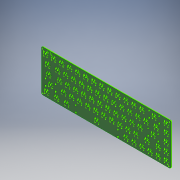
# Autodesk Inventor part: 60pc_pcb.kicad_pcb_Outline
Saved by Autodesk Inventor 2018 (Build 220112000, 112)
## iProperties
Created: 2018-02-01
Part Number: 60pc_pcb.kicad_pcb_Outline
Material: Generic
Document SubType Name: Modeling
Designer: ConnorDevitt
Density: 1 g/cm^3
Appearance: Board Outline
Author: ConnorDevitt
Autodesk Inventor part; units mm, degrees
(part 1 of 2)
ref_plane "YZ Plane" through (0, 0, 0) normal (1, 0, 0) x (0, 1, 0)
ref_plane "XZ Plane" through (0, 0, 0) normal (0, 1, 0) x (-1, 0, 0)
ref_plane "XY Plane" through (0, 0, 0) normal (0, 0, 1) x (1, 0, 0)
sketch "Sketch1" plane through (0, 0, 0) normal (0, 0, 1) x (1, 0, 0)
  arc A0 (77.75, -126.75) -> (81.75, -130.75) centre (81.75, -126.75) ccw
  line L0 (81.75, -130.75) -> (380.25, -130.75)
  arc A1 (380.25, -130.75) -> (384.25, -126.75) centre (380.25, -126.75) ccw
  line L1 (384.25, -126.75) -> (384.25, -35.25)
  arc A2 (384.25, -35.25) -> (381.5, -32.5) centre (381.5, -35.25) ccw
  line L2 (381.5, -32.5) -> (80.5, -32.5)
  arc A3 (80.5, -32.5) -> (77.75, -35.25) centre (80.5, -35.25) ccw
  line L3 (77.75, -35.25) -> (77.75, -126.75)
  line L4 (104.8123, -39.2267) -> (104.0014, -40.6866)
  arc A4 (102.6902, -39.9583) -> (104.0014, -40.6866) centre (103.3458, -40.3225) ccw
  line L5 (102.6902, -39.9583) -> (103.5011, -38.4984)
  arc A5 (104.8123, -39.2267) -> (103.5011, -38.4984) centre (104.1567, -38.8625) ccw
  line L6 (110.4442, -37.8342) -> (110.4048, -38.4128)
  arc A6 (108.9083, -38.3108) -> (110.4048, -38.4128) centre (109.6565, -38.3618) ccw
  line L7 (108.9083, -38.3108) -> (108.9477, -37.7322)
  arc A7 (110.4442, -37.8342) -> (108.9477, -37.7322) centre (109.696, -37.7832) ccw
  line L8 (94.49, -34.45) -> (94.49, -36.95)
  arc A8 (93.79, -36.95) -> (94.49, -36.95) centre (94.14, -36.95) ccw
  line L9 (93.79, -36.95) -> (93.79, -34.45)
  arc A9 (94.49, -34.45) -> (93.79, -34.45) centre (94.14, -34.45) ccw
  line L10 (101.79, -34.45) -> (101.79, -36.95)
  arc A10 (101.09, -36.95) -> (101.79, -36.95) centre (101.44, -36.95) ccw
  line L11 (101.09, -36.95) -> (101.09, -34.45)
  arc A11 (101.79, -34.45) -> (101.09, -34.45) centre (101.44, -34.45) ccw
  line L12 (85.7623, -39.2267) -> (84.9514, -40.6866)
  arc A12 (83.6402, -39.9583) -> (84.9514, -40.6866) centre (84.2958, -40.3225) ccw
  line L13 (83.6402, -39.9583) -> (84.4511, -38.4984)
  arc A13 (85.7623, -39.2267) -> (84.4511, -38.4984) centre (85.1067, -38.8625) ccw
  line L14 (91.3942, -37.8342) -> (91.3548, -38.4128)
  arc A14 (89.8583, -38.3108) -> (91.3548, -38.4128) centre (90.6065, -38.3618) ccw
  line L15 (89.8583, -38.3108) -> (89.8977, -37.7322)
  arc A15 (91.3942, -37.8342) -> (89.8977, -37.7322) centre (90.646, -37.7832) ccw
  line L16 (90.5249, -58.2767) -> (89.7139, -59.7366)
  arc A16 (88.4027, -59.0083) -> (89.7139, -59.7366) centre (89.0583, -59.3725) ccw
  line L17 (88.4027, -59.0083) -> (89.2136, -57.5484)
  arc A17 (90.5249, -58.2767) -> (89.2136, -57.5484) centre (89.8692, -57.9125) ccw
  line L18 (96.1567, -56.8842) -> (96.1173, -57.4628)
  arc A18 (94.6208, -57.3608) -> (96.1173, -57.4628) centre (95.369, -57.4118) ccw
  line L19 (94.6208, -57.3608) -> (94.6602, -56.7822)
  arc A19 (96.1567, -56.8842) -> (94.6602, -56.7822) centre (95.4085, -56.8332) ccw
  line L20 (92.9061, -77.3267) -> (92.0952, -78.7866)
  arc A20 (90.7839, -78.0583) -> (92.0952, -78.7866) centre (91.4395, -78.4225) ccw
  line L21 (90.7839, -78.0583) -> (91.5948, -76.5984)
  arc A21 (92.9061, -77.3267) -> (91.5948, -76.5984) centre (92.2505, -76.9625) ccw
  line L22 (98.538, -75.9342) -> (98.4985, -76.5128)
  arc A22 (97.002, -76.4108) -> (98.4985, -76.5128) centre (97.7503, -76.4618) ccw
  line L23 (97.002, -76.4108) -> (97.0415, -75.8322)
  arc A23 (98.538, -75.9342) -> (97.0415, -75.8322) centre (97.7897, -75.8832) ccw
  line L24 (97.6686, -96.3767) -> (96.8577, -97.8366)
  arc A24 (95.5464, -97.1083) -> (96.8577, -97.8366) centre (96.202, -97.4725) ccw
  line L25 (95.5464, -97.1083) -> (96.3573, -95.6484)
  arc A25 (97.6686, -96.3767) -> (96.3573, -95.6484) centre (97.013, -96.0125) ccw
  line L26 (103.3005, -94.9842) -> (103.261, -95.5628)
  arc A26 (101.7645, -95.4608) -> (103.261, -95.5628) centre (102.5128, -95.5118) ccw
  line L27 (101.7645, -95.4608) -> (101.804, -94.8822)
  arc A27 (103.3005, -94.9842) -> (101.804, -94.8822) centre (102.5522, -94.9332) ccw
  line L28 (88.1436, -115.4267) -> (87.3327, -116.8866)
  arc A28 (86.0214, -116.1583) -> (87.3327, -116.8866) centre (86.677, -116.5225) ccw
  line L29 (86.0214, -116.1583) -> (86.8323, -114.6984)
  arc A29 (88.1436, -115.4267) -> (86.8323, -114.6984) centre (87.488, -115.0625) ccw
  line L30 (93.7755, -114.0342) -> (93.736, -114.6128)
  arc A30 (92.2395, -114.5108) -> (93.736, -114.6128) centre (92.9878, -114.5618) ccw
  line L31 (92.2395, -114.5108) -> (92.279, -113.9322)
  arc A31 (93.7755, -114.0342) -> (92.279, -113.9322) centre (93.0272, -113.9832) ccw
  line L32 (114.3374, -58.2767) -> (113.5264, -59.7366)
  arc A32 (112.2151, -59.0083) -> (113.5264, -59.7366) centre (112.8708, -59.3725) ccw
  line L33 (112.2151, -59.0083) -> (113.0261, -57.5484)
  arc A33 (114.3374, -58.2767) -> (113.0261, -57.5484) centre (113.6817, -57.9125) ccw
  line L34 (119.9692, -56.8842) -> (119.9298, -57.4628)
  arc A34 (118.4333, -57.3608) -> (119.9298, -57.4628) centre (119.1815, -57.4118) ccw
  line L35 (118.4333, -57.3608) -> (118.4727, -56.7822)
  arc A35 (119.9692, -56.8842) -> (118.4727, -56.7822) centre (119.221, -56.8332) ccw
  line L36 (119.0999, -77.3267) -> (118.2889, -78.7866)
  arc A36 (116.9777, -78.0583) -> (118.2889, -78.7866) centre (117.6333, -78.4225) ccw
  line L37 (116.9777, -78.0583) -> (117.7886, -76.5984)
  arc A37 (119.0999, -77.3267) -> (117.7886, -76.5984) centre (118.4442, -76.9625) ccw
  line L38 (124.7317, -75.9342) -> (124.6923, -76.5128)
  arc A38 (123.1958, -76.4108) -> (124.6923, -76.5128) centre (123.944, -76.4618) ccw
  line L39 (123.1958, -76.4108) -> (123.2352, -75.8322)
  arc A39 (124.7317, -75.9342) -> (123.2352, -75.8322) centre (123.9835, -75.8832) ccw
  line L40 (128.6249, -96.3767) -> (127.8139, -97.8366)
  arc A40 (126.5027, -97.1083) -> (127.8139, -97.8366) centre (127.1583, -97.4725) ccw
  line L41 (126.5027, -97.1083) -> (127.3136, -95.6484)
  arc A41 (128.6249, -96.3767) -> (127.3136, -95.6484) centre (127.9692, -96.0125) ccw
  line L42 (134.2567, -94.9842) -> (134.2173, -95.5628)
  arc A42 (132.7208, -95.4608) -> (134.2173, -95.5628) centre (133.469, -95.5118) ccw
  line L43 (132.7208, -95.4608) -> (132.7602, -94.8822)
  arc A43 (134.2567, -94.9842) -> (132.7602, -94.8822) centre (133.5085, -94.9332) ccw
  line L44 (111.9561, -115.4267) -> (111.1452, -116.8866)
  arc A44 (109.8339, -116.1583) -> (111.1452, -116.8866) centre (110.4895, -116.5225) ccw
  line L45 (109.8339, -116.1583) -> (110.6448, -114.6984)
  arc A45 (111.9561, -115.4267) -> (110.6448, -114.6984) centre (111.3005, -115.0625) ccw
  line L46 (117.588, -114.0342) -> (117.5485, -114.6128)
  arc A46 (116.052, -114.5108) -> (117.5485, -114.6128) centre (116.8003, -114.5618) ccw
  line L47 (116.052, -114.5108) -> (116.0915, -113.9322)
  arc A47 (117.588, -114.0342) -> (116.0915, -113.9322) centre (116.8397, -113.9832) ccw
  line L48 (135.7686, -115.4267) -> (134.9577, -116.8866)
  arc A48 (133.6464, -116.1583) -> (134.9577, -116.8866) centre (134.302, -116.5225) ccw
  line L49 (133.6464, -116.1583) -> (134.4573, -114.6984)
  arc A49 (135.7686, -115.4267) -> (134.4573, -114.6984) centre (135.113, -115.0625) ccw
  line L50 (141.4005, -114.0342) -> (141.361, -114.6128)
  arc A50 (139.8645, -114.5108) -> (141.361, -114.6128) centre (140.6128, -114.5618) ccw
  line L51 (139.8645, -114.5108) -> (139.904, -113.9322)
  arc A51 (141.4005, -114.0342) -> (139.904, -113.9322) centre (140.6522, -113.9832) ccw
  line L52 (123.8624, -39.2267) -> (123.0514, -40.6866)
  arc A52 (121.7401, -39.9583) -> (123.0514, -40.6866) centre (122.3958, -40.3225) ccw
  line L53 (121.7401, -39.9583) -> (122.5511, -38.4984)
  arc A53 (123.8624, -39.2267) -> (122.5511, -38.4984) centre (123.2067, -38.8625) ccw
  line L54 (129.4942, -37.8342) -> (129.4548, -38.4128)
  arc A54 (127.9583, -38.3108) -> (129.4548, -38.4128) centre (128.7065, -38.3618) ccw
  line L55 (127.9583, -38.3108) -> (127.9977, -37.7322)
  arc A55 (129.4942, -37.8342) -> (127.9977, -37.7322) centre (128.746, -37.7832) ccw
  line L56 (133.3873, -58.2767) -> (132.5764, -59.7366)
  arc A56 (131.2652, -59.0083) -> (132.5764, -59.7366) centre (131.9208, -59.3725) ccw
  line L57 (131.2652, -59.0083) -> (132.0761, -57.5484)
  arc A57 (133.3873, -58.2767) -> (132.0761, -57.5484) centre (132.7317, -57.9125) ccw
  line L58 (139.0192, -56.8842) -> (138.9798, -57.4628)
  arc A58 (137.4833, -57.3608) -> (138.9798, -57.4628) centre (138.2315, -57.4118) ccw
  line L59 (137.4833, -57.3608) -> (137.5227, -56.7822)
  arc A59 (139.0192, -56.8842) -> (137.5227, -56.7822) centre (138.271, -56.8332) ccw
  line L60 (138.1499, -77.3267) -> (137.3389, -78.7866)
  arc A60 (136.0276, -78.0583) -> (137.3389, -78.7866) centre (136.6833, -78.4225) ccw
  line L61 (136.0276, -78.0583) -> (136.8386, -76.5984)
  arc A61 (138.1499, -77.3267) -> (136.8386, -76.5984) centre (137.4942, -76.9625) ccw
  line L62 (143.7817, -75.9342) -> (143.7423, -76.5128)
  arc A62 (142.2458, -76.4108) -> (143.7423, -76.5128) centre (142.994, -76.4618) ccw
  line L63 (142.2458, -76.4108) -> (142.2852, -75.8322)
  arc A63 (143.7817, -75.9342) -> (142.2852, -75.8322) centre (143.0335, -75.8832) ccw
  line L64 (147.6748, -96.3767) -> (146.8639, -97.8366)
  arc A64 (145.5526, -97.1083) -> (146.8639, -97.8366) centre (146.2083, -97.4725) ccw
  line L65 (145.5526, -97.1083) -> (146.3636, -95.6484)
  arc A65 (147.6748, -96.3767) -> (146.3636, -95.6484) centre (147.0192, -96.0125) ccw
  line L66 (153.3067, -94.9842) -> (153.2673, -95.5628)
  arc A66 (151.7708, -95.4608) -> (153.2673, -95.5628) centre (152.519, -95.5118) ccw
  line L67 (151.7708, -95.4608) -> (151.8102, -94.8822)
  arc A67 (153.3067, -94.9842) -> (151.8102, -94.8822) centre (152.5585, -94.9332) ccw
  line L68 (142.9124, -39.2267) -> (142.1014, -40.6866)
  arc A68 (140.7902, -39.9583) -> (142.1014, -40.6866) centre (141.4458, -40.3225) ccw
  line L69 (140.7902, -39.9583) -> (141.6011, -38.4984)
  arc A69 (142.9124, -39.2267) -> (141.6011, -38.4984) centre (142.2567, -38.8625) ccw
  line L70 (148.5442, -37.8342) -> (148.5048, -38.4128)
  arc A70 (147.0083, -38.3108) -> (148.5048, -38.4128) centre (147.7565, -38.3618) ccw
  line L71 (147.0083, -38.3108) -> (147.0477, -37.7322)
  arc A71 (148.5442, -37.8342) -> (147.0477, -37.7322) centre (147.796, -37.7832) ccw
  line L72 (152.4374, -58.2767) -> (151.6264, -59.7366)
  arc A72 (150.3151, -59.0083) -> (151.6264, -59.7366) centre (150.9708, -59.3725) ccw
  line L73 (150.3151, -59.0083) -> (151.1261, -57.5484)
  arc A73 (152.4374, -58.2767) -> (151.1261, -57.5484) centre (151.7817, -57.9125) ccw
  line L74 (158.0692, -56.8842) -> (158.0298, -57.4628)
  arc A74 (156.5333, -57.3608) -> (158.0298, -57.4628) centre (157.2815, -57.4118) ccw
  line L75 (156.5333, -57.3608) -> (156.5727, -56.7822)
  arc A75 (158.0692, -56.8842) -> (156.5727, -56.7822) centre (157.321, -56.8332) ccw
  line L76 (157.1999, -77.3267) -> (156.3889, -78.7866)
  arc A76 (155.0777, -78.0583) -> (156.3889, -78.7866) centre (155.7333, -78.4225) ccw
  line L77 (155.0777, -78.0583) -> (155.8886, -76.5984)
  arc A77 (157.1999, -77.3267) -> (155.8886, -76.5984) centre (156.5442, -76.9625) ccw
  line L78 (162.8317, -75.9342) -> (162.7923, -76.5128)
  arc A78 (161.2958, -76.4108) -> (162.7923, -76.5128) centre (162.044, -76.4618) ccw
  line L79 (161.2958, -76.4108) -> (161.3352, -75.8322)
  arc A79 (162.8317, -75.9342) -> (161.3352, -75.8322) centre (162.0835, -75.8832) ccw
  line L80 (166.7249, -96.3767) -> (165.9139, -97.8366)
  arc A80 (164.6027, -97.1083) -> (165.9139, -97.8366) centre (165.2583, -97.4725) ccw
  line L81 (164.6027, -97.1083) -> (165.4136, -95.6484)
  arc A81 (166.7249, -96.3767) -> (165.4136, -95.6484) centre (166.0692, -96.0125) ccw
  line L82 (172.3567, -94.9842) -> (172.3173, -95.5628)
  arc A82 (170.8208, -95.4608) -> (172.3173, -95.5628) centre (171.569, -95.5118) ccw
  line L83 (170.8208, -95.4608) -> (170.8602, -94.8822)
  arc A83 (172.3567, -94.9842) -> (170.8602, -94.8822) centre (171.6085, -94.9332) ccw
  line L84 (161.9623, -39.2267) -> (161.1514, -40.6866)
  arc A84 (159.8401, -39.9583) -> (161.1514, -40.6866) centre (160.4958, -40.3225) ccw
  line L85 (159.8401, -39.9583) -> (160.6511, -38.4984)
  arc A85 (161.9623, -39.2267) -> (160.6511, -38.4984) centre (161.3067, -38.8625) ccw
  line L86 (167.5942, -37.8342) -> (167.5548, -38.4128)
  arc A86 (166.0583, -38.3108) -> (167.5548, -38.4128) centre (166.8065, -38.3618) ccw
  line L87 (166.0583, -38.3108) -> (166.0977, -37.7322)
  arc A87 (167.5942, -37.8342) -> (166.0977, -37.7322) centre (166.846, -37.7832) ccw
  line L88 (171.4873, -58.2767) -> (170.6764, -59.7366)
  arc A88 (169.3651, -59.0083) -> (170.6764, -59.7366) centre (170.0208, -59.3725) ccw
  line L89 (169.3651, -59.0083) -> (170.1761, -57.5484)
  arc A89 (171.4873, -58.2767) -> (170.1761, -57.5484) centre (170.8317, -57.9125) ccw
  line L90 (177.1192, -56.8842) -> (177.0798, -57.4628)
  arc A90 (175.5833, -57.3608) -> (177.0798, -57.4628) centre (176.3315, -57.4118) ccw
  line L91 (175.5833, -57.3608) -> (175.6227, -56.7822)
  arc A91 (177.1192, -56.8842) -> (175.6227, -56.7822) centre (176.371, -56.8332) ccw
  line L92 (176.2499, -77.3267) -> (175.4389, -78.7866)
  arc A92 (174.1277, -78.0583) -> (175.4389, -78.7866) centre (174.7833, -78.4225) ccw
  line L93 (174.1277, -78.0583) -> (174.9386, -76.5984)
  arc A93 (176.2499, -77.3267) -> (174.9386, -76.5984) centre (175.5942, -76.9625) ccw
  line L94 (181.8817, -75.9342) -> (181.8423, -76.5128)
  arc A94 (180.3458, -76.4108) -> (181.8423, -76.5128) centre (181.094, -76.4618) ccw
  line L95 (180.3458, -76.4108) -> (180.3852, -75.8322)
  arc A95 (181.8817, -75.9342) -> (180.3852, -75.8322) centre (181.1335, -75.8832) ccw
  line L96 (185.7748, -96.3767) -> (184.9639, -97.8366)
  arc A96 (183.6526, -97.1083) -> (184.9639, -97.8366) centre (184.3083, -97.4725) ccw
  line L97 (183.6526, -97.1083) -> (184.4636, -95.6484)
  arc A97 (185.7748, -96.3767) -> (184.4636, -95.6484) centre (185.1192, -96.0125) ccw
  line L98 (191.4067, -94.9842) -> (191.3673, -95.5628)
  arc A98 (189.8708, -95.4608) -> (191.3673, -95.5628) centre (190.619, -95.5118) ccw
  line L99 (189.8708, -95.4608) -> (189.9102, -94.8822)
  arc A99 (191.4067, -94.9842) -> (189.9102, -94.8822) centre (190.6585, -94.9332) ccw
  line L100 (181.0123, -39.2267) -> (180.2014, -40.6866)
  arc A100 (178.8902, -39.9583) -> (180.2014, -40.6866) centre (179.5458, -40.3225) ccw
  line L101 (178.8902, -39.9583) -> (179.7011, -38.4984)
  arc A101 (181.0123, -39.2267) -> (179.7011, -38.4984) centre (180.3567, -38.8625) ccw
  line L102 (186.6442, -37.8342) -> (186.6048, -38.4128)
  arc A102 (185.1083, -38.3108) -> (186.6048, -38.4128) centre (185.8565, -38.3618) ccw
  line L103 (185.1083, -38.3108) -> (185.1477, -37.7322)
  arc A103 (186.6442, -37.8342) -> (185.1477, -37.7322) centre (185.896, -37.7832) ccw
  line L104 (190.5374, -58.2767) -> (189.7264, -59.7366)
  arc A104 (188.4152, -59.0083) -> (189.7264, -59.7366) centre (189.0708, -59.3725) ccw
  line L105 (188.4152, -59.0083) -> (189.2261, -57.5484)
  arc A105 (190.5374, -58.2767) -> (189.2261, -57.5484) centre (189.8817, -57.9125) ccw
  line L106 (196.1692, -56.8842) -> (196.1298, -57.4628)
  arc A106 (194.6333, -57.3608) -> (196.1298, -57.4628) centre (195.3815, -57.4118) ccw
  line L107 (194.6333, -57.3608) -> (194.6727, -56.7822)
  arc A107 (196.1692, -56.8842) -> (194.6727, -56.7822) centre (195.421, -56.8332) ccw
  line L108 (195.2998, -77.3267) -> (194.4889, -78.7866)
  arc A108 (193.1777, -78.0583) -> (194.4889, -78.7866) centre (193.8333, -78.4225) ccw
  line L109 (193.1777, -78.0583) -> (193.9886, -76.5984)
  arc A109 (195.2998, -77.3267) -> (193.9886, -76.5984) centre (194.6442, -76.9625) ccw
  line L110 (200.9317, -75.9342) -> (200.8923, -76.5128)
  arc A110 (199.3958, -76.4108) -> (200.8923, -76.5128) centre (200.144, -76.4618) ccw
  line L111 (199.3958, -76.4108) -> (199.4352, -75.8322)
  arc A111 (200.9317, -75.9342) -> (199.4352, -75.8322) centre (200.1835, -75.8832) ccw
  line L112 (204.8248, -96.3767) -> (204.0139, -97.8366)
  arc A112 (202.7027, -97.1083) -> (204.0139, -97.8366) centre (203.3583, -97.4725) ccw
  line L113 (202.7027, -97.1083) -> (203.5136, -95.6484)
  arc A113 (204.8248, -96.3767) -> (203.5136, -95.6484) centre (204.1692, -96.0125) ccw
  line L114 (210.4567, -94.9842) -> (210.4173, -95.5628)
  arc A114 (208.9208, -95.4608) -> (210.4173, -95.5628) centre (209.669, -95.5118) ccw
  line L115 (208.9208, -95.4608) -> (208.9602, -94.8822)
  arc A115 (210.4567, -94.9842) -> (208.9602, -94.8822) centre (209.7085, -94.9332) ccw
  line L116 (200.0624, -39.2267) -> (199.2514, -40.6866)
  arc A116 (197.9402, -39.9583) -> (199.2514, -40.6866) centre (198.5958, -40.3225) ccw
  line L117 (197.9402, -39.9583) -> (198.7511, -38.4984)
  arc A117 (200.0624, -39.2267) -> (198.7511, -38.4984) centre (199.4067, -38.8625) ccw
  line L118 (205.6942, -37.8342) -> (205.6548, -38.4128)
  arc A118 (204.1583, -38.3108) -> (205.6548, -38.4128) centre (204.9065, -38.3618) ccw
  line L119 (204.1583, -38.3108) -> (204.1977, -37.7322)
  arc A119 (205.6942, -37.8342) -> (204.1977, -37.7322) centre (204.946, -37.7832) ccw
  line L120 (209.5874, -58.2767) -> (208.7764, -59.7366)
  arc A120 (207.4652, -59.0083) -> (208.7764, -59.7366) centre (208.1208, -59.3725) ccw
  line L121 (207.4652, -59.0083) -> (208.2761, -57.5484)
  arc A121 (209.5874, -58.2767) -> (208.2761, -57.5484) centre (208.9317, -57.9125) ccw
  line L122 (215.2192, -56.8842) -> (215.1798, -57.4628)
  arc A122 (213.6833, -57.3608) -> (215.1798, -57.4628) centre (214.4315, -57.4118) ccw
  line L123 (213.6833, -57.3608) -> (213.7227, -56.7822)
  arc A123 (215.2192, -56.8842) -> (213.7227, -56.7822) centre (214.471, -56.8332) ccw
  line L124 (214.3499, -77.3267) -> (213.5389, -78.7866)
  arc A124 (212.2277, -78.0583) -> (213.5389, -78.7866) centre (212.8833, -78.4225) ccw
  line L125 (212.2277, -78.0583) -> (213.0386, -76.5984)
  arc A125 (214.3499, -77.3267) -> (213.0386, -76.5984) centre (213.6942, -76.9625) ccw
  line L126 (219.9817, -75.9342) -> (219.9423, -76.5128)
  arc A126 (218.4458, -76.4108) -> (219.9423, -76.5128) centre (219.194, -76.4618) ccw
  line L127 (218.4458, -76.4108) -> (218.4852, -75.8322)
  arc A127 (219.9817, -75.9342) -> (218.4852, -75.8322) centre (219.2335, -75.8832) ccw
  line L128 (223.8749, -96.3767) -> (223.0639, -97.8366)
  arc A128 (221.7526, -97.1083) -> (223.0639, -97.8366) centre (222.4083, -97.4725) ccw
  line L129 (221.7526, -97.1083) -> (222.5636, -95.6484)
  arc A129 (223.8749, -96.3767) -> (222.5636, -95.6484) centre (223.2192, -96.0125) ccw
  line L130 (229.5067, -94.9842) -> (229.4673, -95.5628)
  arc A130 (227.9708, -95.4608) -> (229.4673, -95.5628) centre (228.719, -95.5118) ccw
  line L131 (227.9708, -95.4608) -> (228.0102, -94.8822)
  arc A131 (229.5067, -94.9842) -> (228.0102, -94.8822) centre (228.7585, -94.9332) ccw
  line L132 (207.2061, -115.4267) -> (206.3952, -116.8866)
  arc A132 (205.0839, -116.1583) -> (206.3952, -116.8866) centre (205.7395, -116.5225) ccw
  line L133 (205.0839, -116.1583) -> (205.8948, -114.6984)
  arc A133 (207.2061, -115.4267) -> (205.8948, -114.6984) centre (206.5505, -115.0625) ccw
  line L134 (212.838, -114.0342) -> (212.7985, -114.6128)
  arc A134 (211.302, -114.5108) -> (212.7985, -114.6128) centre (212.0503, -114.5618) ccw
  line L135 (211.302, -114.5108) -> (211.3415, -113.9322)
  arc A135 (212.838, -114.0342) -> (211.3415, -113.9322) centre (212.0897, -113.9832) ccw
  line L136 (219.1124, -39.2267) -> (218.3014, -40.6866)
  arc A136 (216.9902, -39.9583) -> (218.3014, -40.6866) centre (217.6458, -40.3225) ccw
  line L137 (216.9902, -39.9583) -> (217.8011, -38.4984)
  arc A137 (219.1124, -39.2267) -> (217.8011, -38.4984) centre (218.4567, -38.8625) ccw
  line L138 (224.7442, -37.8342) -> (224.7048, -38.4128)
  arc A138 (223.2083, -38.3108) -> (224.7048, -38.4128) centre (223.9565, -38.3618) ccw
  line L139 (223.2083, -38.3108) -> (223.2477, -37.7322)
  arc A139 (224.7442, -37.8342) -> (223.2477, -37.7322) centre (223.996, -37.7832) ccw
  line L140 (228.6374, -58.2767) -> (227.8264, -59.7366)
  arc A140 (226.5152, -59.0083) -> (227.8264, -59.7366) centre (227.1708, -59.3725) ccw
  line L141 (226.5152, -59.0083) -> (227.3261, -57.5484)
  arc A141 (228.6374, -58.2767) -> (227.3261, -57.5484) centre (227.9817, -57.9125) ccw
  line L142 (234.2692, -56.8842) -> (234.2298, -57.4628)
  arc A142 (232.7333, -57.3608) -> (234.2298, -57.4628) centre (233.4815, -57.4118) ccw
  line L143 (232.7333, -57.3608) -> (232.7727, -56.7822)
  arc A143 (234.2692, -56.8842) -> (232.7727, -56.7822) centre (233.521, -56.8332) ccw
  line L144 (233.3998, -77.3267) -> (232.5889, -78.7866)
  arc A144 (231.2776, -78.0583) -> (232.5889, -78.7866) centre (231.9333, -78.4225) ccw
  line L145 (231.2776, -78.0583) -> (232.0886, -76.5984)
  arc A145 (233.3998, -77.3267) -> (232.0886, -76.5984) centre (232.7442, -76.9625) ccw
  line L146 (239.0317, -75.9342) -> (238.9923, -76.5128)
  arc A146 (237.4958, -76.4108) -> (238.9923, -76.5128) centre (238.244, -76.4618) ccw
  line L147 (237.4958, -76.4108) -> (237.5352, -75.8322)
  arc A147 (239.0317, -75.9342) -> (237.5352, -75.8322) centre (238.2835, -75.8832) ccw
  line L148 (242.9248, -96.3767) -> (242.1139, -97.8366)
  arc A148 (240.8026, -97.1083) -> (242.1139, -97.8366) centre (241.4583, -97.4725) ccw
  line L149 (240.8026, -97.1083) -> (241.6136, -95.6484)
  arc A149 (242.9248, -96.3767) -> (241.6136, -95.6484) centre (242.2692, -96.0125) ccw
  line L150 (248.5567, -94.9842) -> (248.5173, -95.5628)
  arc A150 (247.0208, -95.4608) -> (248.5173, -95.5628) centre (247.769, -95.5118) ccw
  line L151 (247.0208, -95.4608) -> (247.0602, -94.8822)
  arc A151 (248.5567, -94.9842) -> (247.0602, -94.8822) centre (247.8085, -94.9332) ccw
  line L152 (238.1624, -39.2267) -> (237.3514, -40.6866)
  arc A152 (236.0402, -39.9583) -> (237.3514, -40.6866) centre (236.6958, -40.3225) ccw
  line L153 (236.0402, -39.9583) -> (236.8511, -38.4984)
  arc A153 (238.1624, -39.2267) -> (236.8511, -38.4984) centre (237.5067, -38.8625) ccw
  line L154 (243.7942, -37.8342) -> (243.7548, -38.4128)
  arc A154 (242.2583, -38.3108) -> (243.7548, -38.4128) centre (243.0065, -38.3618) ccw
  line L155 (242.2583, -38.3108) -> (242.2977, -37.7322)
  arc A155 (243.7942, -37.8342) -> (242.2977, -37.7322) centre (243.046, -37.7832) ccw
  line L156 (247.6874, -58.2767) -> (246.8764, -59.7366)
  arc A156 (245.5652, -59.0083) -> (246.8764, -59.7366) centre (246.2208, -59.3725) ccw
  line L157 (245.5652, -59.0083) -> (246.3761, -57.5484)
  arc A157 (247.6874, -58.2767) -> (246.3761, -57.5484) centre (247.0317, -57.9125) ccw
  line L158 (253.3192, -56.8842) -> (253.2798, -57.4628)
  arc A158 (251.7833, -57.3608) -> (253.2798, -57.4628) centre (252.5315, -57.4118) ccw
  line L159 (251.7833, -57.3608) -> (251.8227, -56.7822)
  arc A159 (253.3192, -56.8842) -> (251.8227, -56.7822) centre (252.571, -56.8332) ccw
  line L160 (252.4498, -77.3267) -> (251.6389, -78.7866)
  arc A160 (250.3277, -78.0583) -> (251.6389, -78.7866) centre (250.9833, -78.4225) ccw
  line L161 (250.3277, -78.0583) -> (251.1386, -76.5984)
  arc A161 (252.4498, -77.3267) -> (251.1386, -76.5984) centre (251.7942, -76.9625) ccw
  line L162 (258.0817, -75.9342) -> (258.0423, -76.5128)
  arc A162 (256.5458, -76.4108) -> (258.0423, -76.5128) centre (257.294, -76.4618) ccw
  line L163 (256.5458, -76.4108) -> (256.5852, -75.8322)
  arc A163 (258.0817, -75.9342) -> (256.5852, -75.8322) centre (257.3335, -75.8832) ccw
  line L164 (261.9749, -96.3767) -> (261.1639, -97.8366)
  arc A164 (259.8526, -97.1083) -> (261.1639, -97.8366) centre (260.5083, -97.4725) ccw
  line L165 (259.8526, -97.1083) -> (260.6636, -95.6484)
  arc A165 (261.9749, -96.3767) -> (260.6636, -95.6484) centre (261.3192, -96.0125) ccw
  line L166 (267.6067, -94.9842) -> (267.5673, -95.5628)
  arc A166 (266.0708, -95.4608) -> (267.5673, -95.5628) centre (266.819, -95.5118) ccw
  line L167 (266.0708, -95.4608) -> (266.1102, -94.8822)
  arc A167 (267.6067, -94.9842) -> (266.1102, -94.8822) centre (266.8585, -94.9332) ccw
  line L168 (257.2124, -39.2267) -> (256.4014, -40.6866)
  arc A168 (255.0902, -39.9583) -> (256.4014, -40.6866) centre (255.7458, -40.3225) ccw
  line L169 (255.0902, -39.9583) -> (255.9011, -38.4984)
  arc A169 (257.2124, -39.2267) -> (255.9011, -38.4984) centre (256.5567, -38.8625) ccw
  line L170 (262.8442, -37.8342) -> (262.8048, -38.4128)
  arc A170 (261.3083, -38.3108) -> (262.8048, -38.4128) centre (262.0565, -38.3618) ccw
  line L171 (261.3083, -38.3108) -> (261.3477, -37.7322)
  arc A171 (262.8442, -37.8342) -> (261.3477, -37.7322) centre (262.096, -37.7832) ccw
  line L172 (266.7373, -58.2767) -> (265.9264, -59.7366)
  arc A172 (264.6152, -59.0083) -> (265.9264, -59.7366) centre (265.2708, -59.3725) ccw
  line L173 (264.6152, -59.0083) -> (265.4261, -57.5484)
  arc A173 (266.7373, -58.2767) -> (265.4261, -57.5484) centre (266.0817, -57.9125) ccw
  line L174 (272.3692, -56.8842) -> (272.3298, -57.4628)
  arc A174 (270.8333, -57.3608) -> (272.3298, -57.4628) centre (271.5815, -57.4118) ccw
  line L175 (270.8333, -57.3608) -> (270.8727, -56.7822)
  arc A175 (272.3692, -56.8842) -> (270.8727, -56.7822) centre (271.621, -56.8332) ccw
  line L176 (271.4999, -77.3267) -> (270.6889, -78.7866)
  arc A176 (269.3777, -78.0583) -> (270.6889, -78.7866) centre (270.0333, -78.4225) ccw
  line L177 (269.3777, -78.0583) -> (270.1886, -76.5984)
  arc A177 (271.4999, -77.3267) -> (270.1886, -76.5984) centre (270.8442, -76.9625) ccw
  line L178 (277.1317, -75.9342) -> (277.0923, -76.5128)
  arc A178 (275.5958, -76.4108) -> (277.0923, -76.5128) centre (276.344, -76.4618) ccw
  line L179 (275.5958, -76.4108) -> (275.6352, -75.8322)
  arc A179 (277.1317, -75.9342) -> (275.6352, -75.8322) centre (276.3835, -75.8832) ccw
  line L180 (281.0249, -96.3767) -> (280.2139, -97.8366)
  arc A180 (278.9026, -97.1083) -> (280.2139, -97.8366) centre (279.5583, -97.4725) ccw
  line L181 (278.9026, -97.1083) -> (279.7136, -95.6484)
  arc A181 (281.0249, -96.3767) -> (279.7136, -95.6484) centre (280.3692, -96.0125) ccw
  line L182 (286.6567, -94.9842) -> (286.6173, -95.5628)
  arc A182 (285.1208, -95.4608) -> (286.6173, -95.5628) centre (285.869, -95.5118) ccw
  line L183 (285.1208, -95.4608) -> (285.1602, -94.8822)
  arc A183 (286.6567, -94.9842) -> (285.1602, -94.8822) centre (285.9085, -94.9332) ccw
  line L184 (276.2624, -39.2267) -> (275.4514, -40.6866)
  arc A184 (274.1402, -39.9583) -> (275.4514, -40.6866) centre (274.7958, -40.3225) ccw
  line L185 (274.1402, -39.9583) -> (274.9511, -38.4984)
  arc A185 (276.2624, -39.2267) -> (274.9511, -38.4984) centre (275.6067, -38.8625) ccw
  line L186 (281.8942, -37.8342) -> (281.8548, -38.4128)
  arc A186 (280.3583, -38.3108) -> (281.8548, -38.4128) centre (281.1065, -38.3618) ccw
  line L187 (280.3583, -38.3108) -> (280.3977, -37.7322)
  arc A187 (281.8942, -37.8342) -> (280.3977, -37.7322) centre (281.146, -37.7832) ccw
  line L188 (285.7874, -58.2767) -> (284.9764, -59.7366)
  arc A188 (283.6651, -59.0083) -> (284.9764, -59.7366) centre (284.3208, -59.3725) ccw
  line L189 (283.6651, -59.0083) -> (284.4761, -57.5484)
  arc A189 (285.7874, -58.2767) -> (284.4761, -57.5484) centre (285.1317, -57.9125) ccw
  line L190 (291.4192, -56.8842) -> (291.3798, -57.4628)
  arc A190 (289.8833, -57.3608) -> (291.3798, -57.4628) centre (290.6315, -57.4118) ccw
  line L191 (289.8833, -57.3608) -> (289.9227, -56.7822)
  arc A191 (291.4192, -56.8842) -> (289.9227, -56.7822) centre (290.671, -56.8332) ccw
  line L192 (290.5498, -77.3267) -> (289.7389, -78.7866)
  arc A192 (288.4277, -78.0583) -> (289.7389, -78.7866) centre (289.0833, -78.4225) ccw
  line L193 (288.4277, -78.0583) -> (289.2386, -76.5984)
  arc A193 (290.5498, -77.3267) -> (289.2386, -76.5984) centre (289.8942, -76.9625) ccw
  line L194 (296.1817, -75.9342) -> (296.1423, -76.5128)
  arc A194 (294.6458, -76.4108) -> (296.1423, -76.5128) centre (295.394, -76.4618) ccw
  line L195 (294.6458, -76.4108) -> (294.6852, -75.8322)
  arc A195 (296.1817, -75.9342) -> (294.6852, -75.8322) centre (295.4335, -75.8832) ccw
  line L196 (300.0749, -96.3767) -> (299.2639, -97.8366)
  arc A196 (297.9527, -97.1083) -> (299.2639, -97.8366) centre (298.6083, -97.4725) ccw
  line L197 (297.9527, -97.1083) -> (298.7636, -95.6484)
  arc A197 (300.0749, -96.3767) -> (298.7636, -95.6484) centre (299.4192, -96.0125) ccw
  line L198 (305.7067, -94.9842) -> (305.6673, -95.5628)
  arc A198 (304.1708, -95.4608) -> (305.6673, -95.5628) centre (304.919, -95.5118) ccw
  line L199 (304.1708, -95.4608) -> (304.2102, -94.8822)
  arc A199 (305.7067, -94.9842) -> (304.2102, -94.8822) centre (304.9585, -94.9332) ccw
  line L200 (276.2624, -115.4267) -> (275.4514, -116.8866)
  arc A200 (274.1402, -116.1583) -> (275.4514, -116.8866) centre (274.7958, -116.5225) ccw
  line L201 (274.1402, -116.1583) -> (274.9511, -114.6984)
  arc A201 (276.2624, -115.4267) -> (274.9511, -114.6984) centre (275.6067, -115.0625) ccw
  line L202 (281.8942, -114.0342) -> (281.8548, -114.6128)
  arc A202 (280.3583, -114.5108) -> (281.8548, -114.6128) centre (281.1065, -114.5618) ccw
  line L203 (280.3583, -114.5108) -> (280.3977, -113.9322)
  arc A203 (281.8942, -114.0342) -> (280.3977, -113.9322) centre (281.146, -113.9832) ccw
  line L204 (295.3123, -39.2267) -> (294.5014, -40.6866)
  arc A204 (293.1902, -39.9583) -> (294.5014, -40.6866) centre (293.8458, -40.3225) ccw
  line L205 (293.1902, -39.9583) -> (294.0011, -38.4984)
  arc A205 (295.3123, -39.2267) -> (294.0011, -38.4984) centre (294.6567, -38.8625) ccw
  line L206 (300.9442, -37.8342) -> (300.9048, -38.4128)
  arc A206 (299.4083, -38.3108) -> (300.9048, -38.4128) centre (300.1565, -38.3618) ccw
  line L207 (299.4083, -38.3108) -> (299.4477, -37.7322)
  arc A207 (300.9442, -37.8342) -> (299.4477, -37.7322) centre (300.196, -37.7832) ccw
  line L208 (304.8374, -58.2767) -> (304.0264, -59.7366)
  arc A208 (302.7151, -59.0083) -> (304.0264, -59.7366) centre (303.3708, -59.3725) ccw
  line L209 (302.7151, -59.0083) -> (303.5261, -57.5484)
  arc A209 (304.8374, -58.2767) -> (303.5261, -57.5484) centre (304.1817, -57.9125) ccw
  line L210 (310.4692, -56.8842) -> (310.4298, -57.4628)
  arc A210 (308.9333, -57.3608) -> (310.4298, -57.4628) centre (309.6815, -57.4118) ccw
  line L211 (308.9333, -57.3608) -> (308.9727, -56.7822)
  arc A211 (310.4692, -56.8842) -> (308.9727, -56.7822) centre (309.721, -56.8332) ccw
  line L212 (309.5999, -77.3267) -> (308.7889, -78.7866)
  arc A212 (307.4777, -78.0583) -> (308.7889, -78.7866) centre (308.1333, -78.4225) ccw
  line L213 (307.4777, -78.0583) -> (308.2886, -76.5984)
  arc A213 (309.5999, -77.3267) -> (308.2886, -76.5984) centre (308.9442, -76.9625) ccw
  line L214 (315.2317, -75.9342) -> (315.1923, -76.5128)
  arc A214 (313.6958, -76.4108) -> (315.1923, -76.5128) centre (314.444, -76.4618) ccw
  line L215 (313.6958, -76.4108) -> (313.7352, -75.8322)
  arc A215 (315.2317, -75.9342) -> (313.7352, -75.8322) centre (314.4835, -75.8832) ccw
  line L216 (295.3123, -115.4267) -> (294.5014, -116.8866)
  arc A216 (293.1902, -116.1583) -> (294.5014, -116.8866) centre (293.8458, -116.5225) ccw
  line L217 (293.1902, -116.1583) -> (294.0011, -114.6984)
  arc A217 (295.3123, -115.4267) -> (294.0011, -114.6984) centre (294.6567, -115.0625) ccw
  line L218 (300.9442, -114.0342) -> (300.9048, -114.6128)
  arc A218 (299.4083, -114.5108) -> (300.9048, -114.6128) centre (300.1565, -114.5618) ccw
  line L219 (299.4083, -114.5108) -> (299.4477, -113.9322)
  arc A219 (300.9442, -114.0342) -> (299.4477, -113.9322) centre (300.196, -113.9832) ccw
  line L220 (314.3623, -39.2267) -> (313.5514, -40.6866)
  arc A220 (312.2402, -39.9583) -> (313.5514, -40.6866) centre (312.8958, -40.3225) ccw
  line L221 (312.2402, -39.9583) -> (313.0511, -38.4984)
  arc A221 (314.3623, -39.2267) -> (313.0511, -38.4984) centre (313.7067, -38.8625) ccw
  line L222 (319.9942, -37.8342) -> (319.9548, -38.4128)
  arc A222 (318.4583, -38.3108) -> (319.9548, -38.4128) centre (319.2065, -38.3618) ccw
  line L223 (318.4583, -38.3108) -> (318.4977, -37.7322)
  arc A223 (319.9942, -37.8342) -> (318.4977, -37.7322) centre (319.246, -37.7832) ccw
  line L224 (323.8874, -58.2767) -> (323.0764, -59.7366)
  arc A224 (321.7652, -59.0083) -> (323.0764, -59.7366) centre (322.4208, -59.3725) ccw
  line L225 (321.7652, -59.0083) -> (322.5761, -57.5484)
  arc A225 (323.8874, -58.2767) -> (322.5761, -57.5484) centre (323.2317, -57.9125) ccw
  line L226 (329.5192, -56.8842) -> (329.4798, -57.4628)
  arc A226 (327.9833, -57.3608) -> (329.4798, -57.4628) centre (328.7315, -57.4118) ccw
  line L227 (327.9833, -57.3608) -> (328.0227, -56.7822)
  arc A227 (329.5192, -56.8842) -> (328.0227, -56.7822) centre (328.771, -56.8332) ccw
  line L228 (340.5561, -77.3267) -> (339.7452, -78.7866)
  arc A228 (338.4339, -78.0583) -> (339.7452, -78.7866) centre (339.0895, -78.4225) ccw
  line L229 (338.4339, -78.0583) -> (339.2448, -76.5984)
  arc A229 (340.5561, -77.3267) -> (339.2448, -76.5984) centre (339.9005, -76.9625) ccw
  line L230 (346.188, -75.9342) -> (346.1485, -76.5128)
  arc A230 (344.652, -76.4108) -> (346.1485, -76.5128) centre (345.4003, -76.4618) ccw
  line L231 (344.652, -76.4108) -> (344.6915, -75.8322)
  arc A231 (346.188, -75.9342) -> (344.6915, -75.8322) centre (345.4397, -75.8832) ccw
  line L232 (352.4624, -96.3767) -> (351.6514, -97.8366)
  arc A232 (350.3402, -97.1083) -> (351.6514, -97.8366) centre (350.9958, -97.4725) ccw
  line L233 (350.3402, -97.1083) -> (351.1511, -95.6484)
  arc A233 (352.4624, -96.3767) -> (351.1511, -95.6484) centre (351.8067, -96.0125) ccw
  line L234 (358.0942, -94.9842) -> (358.0548, -95.5628)
  arc A234 (356.5583, -95.4608) -> (358.0548, -95.5628) centre (357.3065, -95.5118) ccw
  line L235 (356.5583, -95.4608) -> (356.5977, -94.8822)
  arc A235 (358.0942, -94.9842) -> (356.5977, -94.8822) centre (357.346, -94.9332) ccw
  line L236 (314.3623, -115.4267) -> (313.5514, -116.8866)
  arc A236 (312.2402, -116.1583) -> (313.5514, -116.8866) centre (312.8958, -116.5225) ccw
  line L237 (312.2402, -116.1583) -> (313.0511, -114.6984)
  arc A237 (314.3623, -115.4267) -> (313.0511, -114.6984) centre (313.7067, -115.0625) ccw
  line L238 (319.9942, -114.0342) -> (319.9548, -114.6128)
  arc A238 (318.4583, -114.5108) -> (319.9548, -114.6128) centre (319.2065, -114.5618) ccw
  line L239 (318.4583, -114.5108) -> (318.4977, -113.9322)
  arc A239 (319.9942, -114.0342) -> (318.4977, -113.9322) centre (319.246, -113.9832) ccw
  line L240 (342.9373, -39.2267) -> (342.1264, -40.6866)
  arc A240 (340.8152, -39.9583) -> (342.1264, -40.6866) centre (341.4708, -40.3225) ccw
  line L241 (340.8152, -39.9583) -> (341.6261, -38.4984)
  arc A241 (342.9373, -39.2267) -> (341.6261, -38.4984) centre (342.2817, -38.8625) ccw
  line L242 (348.5692, -37.8342) -> (348.5298, -38.4128)
  arc A242 (347.0333, -38.3108) -> (348.5298, -38.4128) centre (347.7815, -38.3618) ccw
  line L243 (347.0333, -38.3108) -> (347.0727, -37.7322)
  arc A243 (348.5692, -37.8342) -> (347.0727, -37.7322) centre (347.821, -37.7832) ccw
  line L244 (347.6999, -58.2767) -> (346.8889, -59.7366)
  arc A244 (345.5777, -59.0083) -> (346.8889, -59.7366) centre (346.2333, -59.3725) ccw
  line L245 (345.5777, -59.0083) -> (346.3886, -57.5484)
  arc A245 (347.6999, -58.2767) -> (346.3886, -57.5484) centre (347.0442, -57.9125) ccw
  line L246 (353.3317, -56.8842) -> (353.2923, -57.4628)
  arc A246 (351.7958, -57.3608) -> (353.2923, -57.4628) centre (352.544, -57.4118) ccw
  line L247 (351.7958, -57.3608) -> (351.8352, -56.7822)
  arc A247 (353.3317, -56.8842) -> (351.8352, -56.7822) centre (352.5835, -56.8332) ccw
  line L248 (371.5124, -77.3267) -> (370.7014, -78.7866)
  arc A248 (369.3902, -78.0583) -> (370.7014, -78.7866) centre (370.0458, -78.4225) ccw
  line L249 (369.3902, -78.0583) -> (370.2011, -76.5984)
  arc A249 (371.5124, -77.3267) -> (370.2011, -76.5984) centre (370.8567, -76.9625) ccw
  line L250 (377.1442, -75.9342) -> (377.1048, -76.5128)
  arc A250 (375.6083, -76.4108) -> (377.1048, -76.5128) centre (376.3565, -76.4618) ccw
  line L251 (375.6083, -76.4108) -> (375.6477, -75.8322)
  arc A251 (377.1442, -75.9342) -> (375.6477, -75.8322) centre (376.396, -75.8832) ccw
  line L252 (371.5124, -96.3767) -> (370.7014, -97.8366)
  arc A252 (369.3902, -97.1083) -> (370.7014, -97.8366) centre (370.0458, -97.4725) ccw
  line L253 (369.3902, -97.1083) -> (370.2011, -95.6484)
  arc A253 (371.5124, -96.3767) -> (370.2011, -95.6484) centre (370.8567, -96.0125) ccw
  line L254 (377.1442, -94.9842) -> (377.1048, -95.5628)
  arc A254 (375.6083, -95.4608) -> (377.1048, -95.5628) centre (376.3565, -95.5118) ccw
  line L255 (375.6083, -95.4608) -> (375.6477, -94.8822)
  arc A255 (377.1442, -94.9842) -> (375.6477, -94.8822) centre (376.396, -94.9332) ccw
  line L256 (352.4624, -115.4267) -> (351.6514, -116.8866)
  arc A256 (350.3402, -116.1583) -> (351.6514, -116.8866) centre (350.9958, -116.5225) ccw
  line L257 (350.3402, -116.1583) -> (351.1511, -114.6984)
  arc A257 (352.4624, -115.4267) -> (351.1511, -114.6984) centre (351.8067, -115.0625) ccw
  line L258 (358.0942, -114.0342) -> (358.0548, -114.6128)
  arc A258 (356.5583, -114.5108) -> (358.0548, -114.6128) centre (357.3065, -114.5618) ccw
  line L259 (356.5583, -114.5108) -> (356.5977, -113.9322)
  arc A259 (358.0942, -114.0342) -> (356.5977, -113.9322) centre (357.346, -113.9832) ccw
  line L260 (371.5124, -39.2267) -> (370.7014, -40.6866)
  arc A260 (369.3902, -39.9583) -> (370.7014, -40.6866) centre (370.0458, -40.3225) ccw
  line L261 (369.3902, -39.9583) -> (370.2011, -38.4984)
  arc A261 (371.5124, -39.2267) -> (370.2011, -38.4984) centre (370.8567, -38.8625) ccw
  line L262 (377.1442, -37.8342) -> (377.1048, -38.4128)
  arc A262 (375.6083, -38.3108) -> (377.1048, -38.4128) centre (376.3565, -38.3618) ccw
  line L263 (375.6083, -38.3108) -> (375.6477, -37.7322)
  arc A263 (377.1442, -37.8342) -> (375.6477, -37.7322) centre (376.396, -37.7832) ccw
  line L264 (371.5124, -58.2767) -> (370.7014, -59.7366)
  arc A264 (369.3902, -59.0083) -> (370.7014, -59.7366) centre (370.0458, -59.3725) ccw
  line L265 (369.3902, -59.0083) -> (370.2011, -57.5484)
  arc A265 (371.5124, -58.2767) -> (370.2011, -57.5484) centre (370.8567, -57.9125) ccw
  line L266 (377.1442, -56.8842) -> (377.1048, -57.4628)
  arc A266 (375.6083, -57.3608) -> (377.1048, -57.4628) centre (376.3565, -57.4118) ccw
  line L267 (375.6083, -57.3608) -> (375.6477, -56.7822)
  arc A267 (377.1442, -56.8842) -> (375.6477, -56.7822) centre (376.396, -56.8332) ccw
  line L268 (371.5124, -115.4267) -> (370.7014, -116.8866)
  arc A268 (369.3902, -116.1583) -> (370.7014, -116.8866) centre (370.0458, -116.5225) ccw
  line L269 (369.3902, -116.1583) -> (370.2011, -114.6984)
  arc A269 (371.5124, -115.4267) -> (370.2011, -114.6984) centre (370.8567, -115.0625) ccw
  line L270 (377.1442, -114.0342) -> (377.1048, -114.6128)
  arc A270 (375.6083, -114.5108) -> (377.1048, -114.6128) centre (376.3565, -114.5618) ccw
  line L271 (375.6083, -114.5108) -> (375.6477, -113.9322)
  arc A271 (377.1442, -114.0342) -> (375.6477, -113.9322) centre (376.396, -113.9832) ccw
  line L272 (333.4124, -115.4267) -> (332.6014, -116.8866)
  arc A272 (331.2902, -116.1583) -> (332.6014, -116.8866) centre (331.9458, -116.5225) ccw
  line L273 (331.2902, -116.1583) -> (332.1011, -114.6984)
  arc A273 (333.4124, -115.4267) -> (332.1011, -114.6984) centre (332.7567, -115.0625) ccw
  line L274 (339.0442, -114.0342) -> (339.0048, -114.6128)
  arc A274 (337.5083, -114.5108) -> (339.0048, -114.6128) centre (338.2565, -114.5618) ccw
  line L275 (337.5083, -114.5108) -> (337.5477, -113.9322)
  arc A275 (339.0442, -114.0342) -> (337.5477, -113.9322) centre (338.296, -113.9832) ccw
  line L276 (326.2686, -96.3767) -> (325.4577, -97.8366)
  arc A276 (324.1464, -97.1083) -> (325.4577, -97.8366) centre (324.802, -97.4725) ccw
  line L277 (324.1464, -97.1083) -> (324.9573, -95.6484)
  arc A277 (326.2686, -96.3767) -> (324.9573, -95.6484) centre (325.613, -96.0125) ccw
  line L278 (331.9005, -94.9842) -> (331.861, -95.5628)
  arc A278 (330.3645, -95.4608) -> (331.861, -95.5628) centre (331.1128, -95.5118) ccw
  line L279 (330.3645, -95.4608) -> (330.404, -94.8822)
  arc A279 (331.9005, -94.9842) -> (330.404, -94.8822) centre (331.1522, -94.9332) ccw
  circle A280 centre (92.0063, -47.625) radius 0.35
  circle A281 centre (84.2062, -47.625) radius 0.35
  circle A282 centre (118.2, -123.825) radius 0.35
  circle A283 centre (110.4, -123.825) radius 0.35
  circle A284 centre (142.0125, -123.825) radius 0.35
  circle A285 centre (134.2125, -123.825) radius 0.35
  circle A286 centre (130.1062, -47.625) radius 0.35
  circle A287 centre (122.3063, -47.625) radius 0.35
  circle A288 centre (139.6312, -66.675) radius 0.35
  circle A289 centre (131.8313, -66.675) radius 0.35
  circle A290 centre (144.3938, -85.725) radius 0.35
  circle A291 centre (136.5938, -85.725) radius 0.35
  circle A292 centre (153.9187, -104.775) radius 0.35
  circle A293 centre (146.1188, -104.775) radius 0.35
  circle A294 centre (149.1562, -47.625) radius 0.35
  circle A295 centre (141.3562, -47.625) radius 0.35
  circle A296 centre (158.6813, -66.675) radius 0.35
  circle A297 centre (150.8812, -66.675) radius 0.35
  circle A298 centre (163.4437, -85.725) radius 0.35
  circle A299 centre (155.6438, -85.725) radius 0.35
  circle A300 centre (172.9688, -104.775) radius 0.35
  circle A301 centre (165.1687, -104.775) radius 0.35
  circle A302 centre (96.7688, -66.675) radius 0.35
  circle A303 centre (88.9688, -66.675) radius 0.35
  circle A304 centre (168.2063, -47.625) radius 0.35
  circle A305 centre (160.4063, -47.625) radius 0.35
  circle A306 centre (177.7312, -66.675) radius 0.35
  circle A307 centre (169.9313, -66.675) radius 0.35
  circle A308 centre (182.4938, -85.725) radius 0.35
  circle A309 centre (174.6937, -85.725) radius 0.35
  circle A310 centre (192.0188, -104.775) radius 0.35
  circle A311 centre (184.2188, -104.775) radius 0.35
  circle A312 centre (187.2563, -47.625) radius 0.35
  circle A313 centre (179.4563, -47.625) radius 0.35
  circle A314 centre (196.7812, -66.675) radius 0.35
  circle A315 centre (188.9812, -66.675) radius 0.35
  circle A316 centre (201.5438, -85.725) radius 0.35
  circle A317 centre (193.7438, -85.725) radius 0.35
  circle A318 centre (211.0688, -104.775) radius 0.35
  circle A319 centre (203.2688, -104.775) radius 0.35
  circle A320 centre (99.15, -85.725) radius 0.35
  circle A321 centre (91.35, -85.725) radius 0.35
  circle A322 centre (206.3063, -47.625) radius 0.35
  circle A323 centre (198.5063, -47.625) radius 0.35
  circle A324 centre (215.8313, -66.675) radius 0.35
  circle A325 centre (208.0312, -66.675) radius 0.35
  circle A326 centre (220.5938, -85.725) radius 0.35
  circle A327 centre (212.7938, -85.725) radius 0.35
  circle A328 centre (230.1188, -104.775) radius 0.35
  circle A329 centre (222.3188, -104.775) radius 0.35
  circle A330 centre (213.45, -123.825) radius 0.35
  circle A331 centre (205.65, -123.825) radius 0.35
  circle A332 centre (225.3562, -47.625) radius 0.35
  circle A333 centre (217.5563, -47.625) radius 0.35
  circle A334 centre (234.8812, -66.675) radius 0.35
  circle A335 centre (227.0813, -66.675) radius 0.35
  circle A336 centre (239.6438, -85.725) radius 0.35
  circle A337 centre (231.8438, -85.725) radius 0.35
  circle A338 centre (249.1688, -104.775) radius 0.35
  circle A339 centre (241.3688, -104.775) radius 0.35
  circle A340 centre (103.9125, -104.775) radius 0.35
  circle A341 centre (96.1125, -104.775) radius 0.35
  circle A342 centre (244.4062, -47.625) radius 0.35
  circle A343 centre (236.6062, -47.625) radius 0.35
  circle A344 centre (253.9313, -66.675) radius 0.35
  circle A345 centre (246.1312, -66.675) radius 0.35
  circle A346 centre (258.6938, -85.725) radius 0.35
  circle A347 centre (250.8938, -85.725) radius 0.35
  circle A348 centre (268.2188, -104.775) radius 0.35
  circle A349 centre (260.4187, -104.775) radius 0.35
  circle A350 centre (263.4563, -47.625) radius 0.35
  circle A351 centre (255.6562, -47.625) radius 0.35
  circle A352 centre (272.9812, -66.675) radius 0.35
  circle A353 centre (265.1812, -66.675) radius 0.35
  circle A354 centre (277.7437, -85.725) radius 0.35
  circle A355 centre (269.9438, -85.725) radius 0.35
  circle A356 centre (287.2688, -104.775) radius 0.35
  circle A357 centre (279.4688, -104.775) radius 0.35
  circle A358 centre (94.3875, -123.825) radius 0.35
  circle A359 centre (86.5875, -123.825) radius 0.35
  circle A360 centre (282.5063, -47.625) radius 0.35
  circle A361 centre (274.7063, -47.625) radius 0.35
  circle A362 centre (292.0312, -66.675) radius 0.35
  circle A363 centre (284.2312, -66.675) radius 0.35
  circle A364 centre (296.7937, -85.725) radius 0.35
  circle A365 centre (288.9937, -85.725) radius 0.35
  circle A366 centre (306.3188, -104.775) radius 0.35
  circle A367 centre (298.5188, -104.775) radius 0.35
  circle A368 centre (282.5063, -123.825) radius 0.35
  circle A369 centre (274.7063, -123.825) radius 0.35
  circle A370 centre (301.5562, -47.625) radius 0.35
  circle A371 centre (293.7563, -47.625) radius 0.35
  circle A372 centre (311.0813, -66.675) radius 0.35
  circle A373 centre (303.2812, -66.675) radius 0.35
  circle A374 centre (315.8438, -85.725) radius 0.35
  circle A375 centre (308.0437, -85.725) radius 0.35
  circle A376 centre (332.5125, -104.775) radius 0.35
  circle A377 centre (324.7125, -104.775) radius 0.35
  circle A378 centre (111.0563, -47.625) radius 0.35
  circle A379 centre (103.2563, -47.625) radius 0.35
  circle A380 centre (301.5562, -123.825) radius 0.35
  circle A381 centre (293.7563, -123.825) radius 0.35
  circle A382 centre (320.6063, -47.625) radius 0.35
  circle A383 centre (312.8062, -47.625) radius 0.35
  circle A384 centre (330.1313, -66.675) radius 0.35
  circle A385 centre (322.3313, -66.675) radius 0.35
  circle A386 centre (346.8, -85.725) radius 0.35
  circle A387 centre (339, -85.725) radius 0.35
  circle A388 centre (358.7063, -104.775) radius 0.35
  circle A389 centre (350.9062, -104.775) radius 0.35
  circle A390 centre (320.6063, -123.825) radius 0.35
  circle A391 centre (312.8062, -123.825) radius 0.35
  circle A392 centre (349.1812, -47.625) radius 0.35
  circle A393 centre (341.3813, -47.625) radius 0.35
  circle A394 centre (353.9438, -66.675) radius 0.35
  circle A395 centre (346.1438, -66.675) radius 0.35
  circle A396 centre (377.7563, -85.725) radius 0.35
  circle A397 centre (369.9563, -85.725) radius 0.35
  circle A398 centre (377.7563, -104.775) radius 0.35
  circle A399 centre (369.9563, -104.775) radius 0.35
  circle A400 centre (120.5813, -66.675) radius 0.35
  circle A401 centre (112.7813, -66.675) radius 0.35
  circle A402 centre (358.7063, -123.825) radius 0.35
  circle A403 centre (350.9062, -123.825) radius 0.35
  circle A404 centre (377.7563, -47.625) radius 0.35
  circle A405 centre (369.9563, -47.625) radius 0.35
  circle A406 centre (377.7563, -66.675) radius 0.35
  circle A407 centre (369.9563, -66.675) radius 0.35
  circle A408 centre (339.6562, -123.825) radius 0.35
  circle A409 centre (331.8563, -123.825) radius 0.35
  circle A410 centre (377.7563, -123.825) radius 0.35
  circle A411 centre (369.9563, -123.825) radius 0.35
  circle A412 centre (125.3438, -85.725) radius 0.35
  circle A413 centre (117.5438, -85.725) radius 0.35
  circle A414 centre (134.8688, -104.775) radius 0.35
  circle A415 centre (127.0688, -104.775) radius 0.35
  circle A416 centre (88.1063, -42.8625) radius 1.994
  circle A417 centre (83.0263, -42.8625) radius 0.851
  circle A418 centre (93.1863, -42.8625) radius 0.851
  circle A419 centre (114.3, -119.0625) radius 1.994
  circle A420 centre (109.22, -119.0625) radius 0.851
  circle A421 centre (119.38, -119.0625) radius 0.851
  circle A422 centre (138.1125, -119.0625) radius 1.994
  circle A423 centre (133.0325, -119.0625) radius 0.851
  circle A424 centre (143.1925, -119.0625) radius 0.851
  circle A425 centre (126.2063, -42.8625) radius 1.994
  circle A426 centre (121.1263, -42.8625) radius 0.851
  circle A427 centre (131.2862, -42.8625) radius 0.851
  circle A428 centre (135.7312, -61.9125) radius 1.994
  circle A429 centre (130.6513, -61.9125) radius 0.851
  circle A430 centre (140.8113, -61.9125) radius 0.851
  circle A431 centre (140.4938, -80.9625) radius 1.994
  circle A432 centre (135.4137, -80.9625) radius 0.851
  circle A433 centre (145.5738, -80.9625) radius 0.851
  circle A434 centre (150.0188, -100.0125) radius 1.994
  circle A435 centre (144.9387, -100.0125) radius 0.851
  circle A436 centre (155.0987, -100.0125) radius 0.851
  circle A437 centre (145.2562, -42.8625) radius 1.994
  circle A438 centre (140.1763, -42.8625) radius 0.851
  circle A439 centre (150.3363, -42.8625) radius 0.851
  circle A440 centre (154.7812, -61.9125) radius 1.994
  circle A441 centre (149.7012, -61.9125) radius 0.851
  circle A442 centre (159.8613, -61.9125) radius 0.851
  circle A443 centre (159.5437, -80.9625) radius 1.994
  circle A444 centre (154.4638, -80.9625) radius 0.851
  circle A445 centre (164.6238, -80.9625) radius 0.851
  circle A446 centre (169.0687, -100.0125) radius 1.994
  circle A447 centre (163.9888, -100.0125) radius 0.851
  circle A448 centre (174.1488, -100.0125) radius 0.851